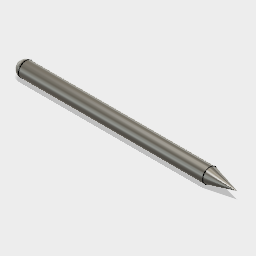
FPROJ_2_LIUYH (Autodesk Fusion 360 design; units mm, degrees)
Autodesk Fusion 360 part; units mm, degrees
cylinder "圆柱体基本要素1" add diameter 8 height 100 placed x (0, 0, -1) y (0, 1, 0) z (1, 0, 0) at (0, 0, 0) makes body 1
sphere "球体基本要素1" add diameter 8 placed x (0, 0, -1) y (0, 1, 0) z (1, 0, 0) at (0, 31.252, 24.8983) separate body makes body 2
move_body "对齐1" bodies 2 to x (1, 0, 0) y (0, 1, 0) z (0, 0, 1) at (0, -31.252, -24.8983)
sketch "草图3" plane through (0, 0, 0) normal (0, 1, 0) x (1, 0, 0)
  line L0 (15, 50) -> (30, 50)
  line L1 (30, 50) -> (30, 47.4986)
  line L2 (30, 47.4986) -> (15, 50)
sketch "草图4" plane through (0, 0, 0) normal (1, 0, 0) x (0, 0, -1)
sketch "草图5" plane through (0, 0, 0) normal (0, 0, 1) x (1, 0, 0)
  line L0 (75, 25) -> (90, 25)
  line L1 (75, 25) -> (75, 29)
  line L2 (90, 25) -> (75, 29)
  dimension "d5" = 4
  measures "d5" distance of L0.start L1.end
revolve "旋转2" add sketch "草图5" angle 360 about axis through (75, 25, 0) along (1, 0, 0) separate body makes body 3
move_body "对齐2" bodies 3 to x (1, 0, 0) y (0, 1, 0) z (0, 0, 1) at (25, -25, 0)
combine "合并1" operation add target body 3 tool bodies 1 2
